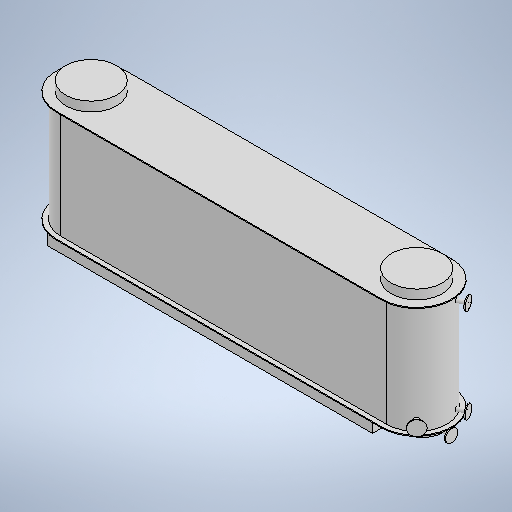
# Autodesk Inventor part: GNG НаOCl tank
Saved by Autodesk Inventor 2025.3 (Build 293356030, 356C)
## iProperties
Created: 2025-09-24
Part Number: GNG НаOCl tank
Material: Generic
Document SubType Name: Modeling
Designer: admin
Density: 1 g/cm^3
Appearance: Default
Mass: 3.1282e+06 g
Surface Area: 160641 cm^2
Volume: 3.1282e+06 cm^3
Author: admin
Autodesk Inventor part; units mm, degrees
sketch "Sketch1" plane through (0, 0, 0) normal (0, 0, 1) x (1, 0, 0)
  line L0 (-1750, 0) -> (1750, 0) construction
  line L1 (-1750, -325) -> (1750, -325)
  line L2 (1750, 325) -> (-1750, 325)
  arc A0 (-1750, 325) -> (-1750, -325) centre (-1750, 0) ccw
  arc A1 (1750, -325) -> (1750, 325) centre (1750, 0) ccw
  point P0 (0, 0)
  point P1 (0, 0)
  dimension "d0" = 3500
  dimension "d1" = 650
  constraints: 8 end point, 4 point on circle, 4 tangent, 2 centre point, 1 coincident, 1 horizontal, 1 midpoint, 1 parallel
  measures "d0" distance of L0.start L0.end
  measures "d1" diameter of A1
extrude "Extrusion1" add sketch "Sketch1" along normal blind 1200
sketch "Sketch2" plane through (0, 0, 1200) normal (0, 0, 1) x (1, 0, 0)
  arc A0 (1750, -325) -> (1750, 325) centre (1750, 0) ccw projected
  line L0 (1750, 325) -> (-1750, 325) projected
  arc A1 (-1750, 325) -> (-1750, -325) centre (-1750, 0) ccw projected
  line L1 (-1750, -325) -> (1750, -325) projected
  line L2 (-1750, 375) -> (1750, 375)
  arc A2 (1750, -375) -> (1750, 375) centre (1750, 0) ccw
  line L3 (1750, -375) -> (-1750, -375)
  arc A3 (-1750, 375) -> (-1750, -375) centre (-1750, 0) ccw
  point P0 (0, 0)
  dimension "d4" = 50
  constraints: 4 end point, 4 point on circle, 2 centre point, 3 other
  measures "d4" distance between parallel lines of L0 L2
extrude "Extrusion2" add sketch "Sketch2" against normal blind 10
sketch "Sketch3" plane through (0, 0, 0) normal (0, 0, -1) x (-1, 0, 0)
  arc A0 (-1750, 325) -> (-1750, -325) centre (-1750, 0) ccw projected
  line L0 (1750, -325) -> (-1750, -325) projected
  arc A1 (1750, -325) -> (1750, 325) centre (1750, 0) ccw projected
  line L1 (-1750, 325) -> (1750, 325) projected
  arc A2 (-1750, 375) -> (-1750, -375) centre (-1750, 0) ccw
  line L2 (-1750, 375) -> (1750, 375)
  arc A3 (1750, -375) -> (1750, 375) centre (1750, 0) ccw
  line L3 (1750, -375) -> (-1750, -375)
  point P0 (0, 0)
  dimension "d7" = 50
  constraints: 4 end point, 4 point on circle, 2 centre point, 3 other
  measures "d7" distance between parallel lines of L0 L3
extrude "Extrusion3" add sketch "Sketch3" against normal blind 10
sketch "Sketch4" plane through (0, 0, 0) normal (0, 0, -1) x (-1, 0, 0)
  circle A0 centre (-1820, 0) radius 200
  arc A1 (-1750, 325) -> (-1750, -325) centre (-1750, 0) ccw projected
  arc A2 (-1750, 325) -> (-1750, -325) centre (-1750, 0) ccw projected
  point P0 (0, 0)
  dimension "d10" = 400
  dimension "d59" = 70
  constraints: 1 centre point, 1 horizontal alignment
  measures "d10" diameter of A0
  measures "d59" distance of A1.centre A0.centre
extrude "Extrusion4" add sketch "Sketch4" along normal blind 100
ref_plane "Work Plane1" through (1750, -325, 0) normal (-1, 0, 0) x (0, 0, 1)
sketch "Sketch5" plane through (1750, -325, 0) normal (-1, 0, 0) x (0, 0, 1)
  line L0 (-100, 525) -> (-100, 125) projected
  line L1 (0, 125) -> (0, 525) projected
  circle A0 centre (-70, 325) radius 20
  point P0 (0, 325)
  point P1 (0, 125)
  point P2 (0, 525)
  point P3 (0, 325)
  dimension "d13" = 40
  dimension "d14" = 30
  constraints: 1 centre point, 1 horizontal alignment, 1 midpoint
  measures "d13" diameter of A0
  measures "d14" distance from line of A0.centre L0
extrude "Extrusion5" add sketch "Sketch5" against normal blind 375
sketch "Sketch6" plane through (2125, 0, -70) normal (1, 0, 0) x (0, 0, -1)
  circle A0 centre (0, 0) radius 20 projected
  circle A1 centre (0, 0) radius 67.5
  line L0 (-70, -375) -> (-70, 375) projected
  line L1 (67.5, 0) -> (67.5, -294.9779)
  point P0 (-70, 0)
  dimension "d18" = 135
  dimension "d40" = 137.5
  constraints: 2 end point, 2 vertical, 1 coincident, 1 horizontal alignment, 2 other
  measures "d40" distance between parallel lines of L1 L0
extrude "Extrusion6" add sketch "Sketch6" against normal blind 10
sketch "Sketch7" plane through (0, 0, 1200) normal (0, 0, 1) x (1, 0, 0)
  line L0 (1750, 375) -> (-1750, 375) projected
  arc A0 (-1750, 375) -> (-1750, -375) centre (-1750, 0) ccw projected
  line L1 (-1750, -375) -> (1750, -375) projected
  arc A1 (1750, -375) -> (1750, 375) centre (1750, 0) ccw projected
  line L2 (1750, 0) -> (2125, 0)
  line L3 (1750, 0) -> (2096.4548, 143.5063)
  line L4 (1750, 0) -> (2015.165, -265.165)
  point P0 (0, 0)
  dimension "d21" = 22.5
  dimension "d23" = 45
  constraints: 6 end point, 3 point on circle
  measures "d21" angle of L2 L3
  measures "d23" angle of L2 L4
ref_plane "Work Plane2" through (2096.4548, 143.5063, 1200) normal (0.9239, 0.3827, 0) x (-0.3827, 0.9239, 0)
ref_plane "Work Plane3" through (2015.165, -265.165, 1200) normal (0.7071, -0.7071, 0) x (0.7071, 0.7071, 0)
sketch "Sketch8" plane through (2096.4548, 143.5063, 1200) normal (0.9239, 0.3827, 0) x (-0.3827, 0.9239, 0)
  line L0 (300.2608, -1190) -> (300.2608, -10) projected
  line L1 (-300.2608, -1190) -> (-300.2608, -10) projected
  circle A0 centre (0, -110) radius 20
  circle A1 centre (0, -1120) radius 20
  line L2 (-300.2608, -1190) -> (300.2608, -1190) projected
  line L3 (300.2608, -10) -> (-300.2608, -10) projected
  point P0 (669.696, -1200)
  point P1 (0, 0)
  point P2 (0, 0)
  point P3 (0, 0)
  dimension "d24" = 40
  constraints: 2 centre point, 2 vertical alignment, 1 equal radius
  measures "d24" diameter of A0
extrude "Extrusion7" add sketch "Sketch8" along normal blind 50 and the other way blind 100 contours A0 | A1
sketch "Sketch9" plane through (2015.165, -265.165, 1200) normal (0.7071, -0.7071, 0) x (0.7071, 0.7071, 0)
  line L0 (229.8097, -1190) -> (229.8097, -10) projected
  line L1 (-229.8097, -1190) -> (-229.8097, -10) projected
  circle A0 centre (0, -1090) radius 31.5
  line L2 (-229.8097, -1190) -> (229.8097, -1190) projected
  line L3 (229.8097, -10) -> (-229.8097, -10) projected
  point P0 (-1237.4369, -1200)
  point P1 (0, 0)
  point P2 (0, 0)
  point P3 (0, 0)
  dimension "d31" = 63
  constraints: 1 centre point, 1 vertical alignment
  measures "d31" diameter of A0
extrude "Extrusion8" add sketch "Sketch9" along normal blind 50 and the other way blind 100 contours A0
sketch "Sketch10" plane through (2050.5204, -300.5204, 110) normal (0.7071, -0.7071, 0) x (-0.7071, -0.7071, 0)
  circle A0 centre (0, 0) radius 31.5 projected
  circle A1 centre (0, 0) radius 80
  point P0 (1237.4369, 110)
  dimension "d37" = 160
  constraints: 1 centre point, 1 coincident
  measures "d37" diameter of A1
extrude "Extrusion9" add sketch "Sketch10" against normal blind 10
sketch "Sketch13" plane through (2142.6488, 162.6405, 80) normal (0.9239, 0.3827, 0) x (0, 0, -1)
  circle A0 centre (0, 0) radius 20 projected
  circle A1 centre (-1010, 0) radius 20 projected
  circle A2 centre (-1010, 0) radius 67.5
  circle A3 centre (0, 0) radius 67.5
  point P0 (80, 669.696)
  dimension "d44" = 135
  dimension "d45" = 135
  constraints: 2 centre point, 2 coincident
  measures "d44" diameter of A2
  measures "d45" diameter of A3
extrude "Extrusion10" add sketch "Sketch13" against normal blind 10
sketch "Sketch14" plane through (0, 0, 1200) normal (0, 0, 1) x (1, 0, 0)
  arc A0 (-1750, 325) -> (-1750, -325) centre (-1750, 0) ccw projected
  circle A1 centre (-1750, 0) radius 275
  arc A2 (1750, -325) -> (1750, 325) centre (1750, 0) ccw projected
  circle A3 centre (1750, 0) radius 275
  point P0 (0, 0)
  dimension "d48" = 550
  dimension "d49" = 550
  constraints: 2 centre point, 2 coincident
  measures "d48" diameter of A1
  measures "d49" diameter of A3
extrude "Extrusion11" add sketch "Sketch14" along normal blind 100
sketch "Sketch15" plane through (0, 0, 0) normal (0, 0, -1) x (-1, 0, 0)
  line L0 (-1550, -175) -> (1950, -175)
  line L1 (1950, -175) -> (1950, -275)
  line L2 (1950, -275) -> (-1550, -275)
  line L3 (-1550, -275) -> (-1550, -175)
  line L4 (-1550, 175) -> (1950, 175)
  line L5 (1950, 175) -> (1950, 275)
  line L6 (1950, 275) -> (-1550, 275)
  line L7 (-1550, 275) -> (-1550, 175)
  line L8 (0, 0) -> (1601.4789, 0)
  line L9 (1750, 375) -> (-1750, 375) projected
  point P0 (200, -275)
  point P1 (0, 375)
  dimension "d52" = 100
  dimension "d53" = 550
  dimension "d58" = 1950
  dimension "d60" = 1550
  constraints: 18 end point, 4 parallel, 3 horizontal, 2 equal length, 2 midpoint, 2 perpendicular, 1 collinear, 1 other
  measures "d52" distance of L0.end L1.end
  measures "d53" distance between parallel lines of L6 L2
  measures "d58" distance from line of L5 L8.start
  measures "d60" horizontal distance of L2.end point (0, 375)
extrude "Extrusion12" add sketch "Sketch15" along normal blind 200
body "Solid1"
